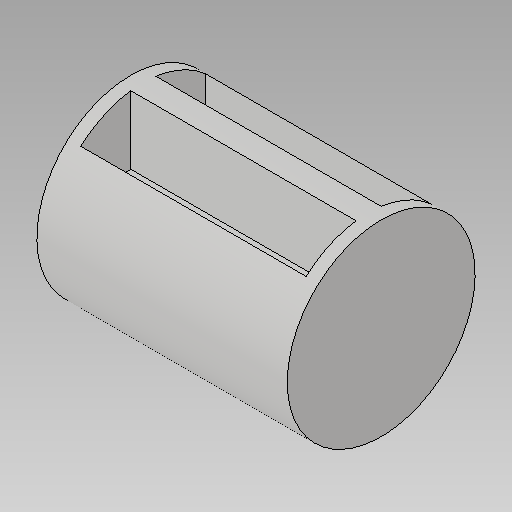
# Autodesk Inventor part: Rounded_beam_body-01
Saved by Autodesk Inventor 2020 (Build 240168000, 168)
## iProperties
Created: 2019-02-05
Part Number: Rounded_beam_body-01
Material: Generic
Document SubType Name: Modeling
Designer: Varga Daniel
Density: 1 g/cm^3
Appearance: Default
Beam_body_length: 10,000 mm
Author: Varga Daniel
Autodesk Inventor part; units mm, degrees
ref_plane "YZ Plane" through (0, 0, 0) normal (1, 0, 0) x (0, 1, 0)
ref_plane "XZ Plane" through (0, 0, 0) normal (0, 1, 0) x (-1, 0, 0)
ref_plane "XY Plane" through (0, 0, 0) normal (0, 0, 1) x (1, 0, 0)
derived "Connector_pin_base.ipt"
sketch "Pin_base_sketch" plane through (0, 0, 0) normal (0, 0, 1) x (1, 0, 0)
  line L0 (0, 0) -> (23.0918, 0) construction
  line L1 (0, 0) -> (0, 6.22) construction
  line L2 (0, 3.75) -> (0.525, 3.75)
  line L3 (0.825, 3.45) -> (0.825, 2.4)
  line L4 (0.825, 2.4) -> (9.225, 2.4)
  line L5 (0, 0) -> (0, 3.75)
  line L6 (0, 0) -> (3.25, 0)
  arc A0 (0.825, 3.45) -> (0.525, 3.75) centre (0.525, 3.45) ccw
  line L7 (0.825, 2.4) -> (0.825, 0.575)
  line L8 (0, 0) -> (-23.0918, 0) construction
  line L9 (9.225, 2.4) -> (9.225, 0.575)
  line L10 (10.025, 2.4) -> (10.025, 2.1865) construction
  line L11 (9.225, 2.4) -> (10.025, 2.4) construction
  line L12 (9.625, 2.4) -> (9.625, 0) construction
  line L13 (10.1291, 2.615) -> (7.4184, 2.615) construction
  line L14 (10.025, 0.575) -> (9.225, 0.575) construction
  line L15 (10.025, 0.575) -> (10.025, 0)
  arc A1 (7.1, 0.575) -> (6.525, 0) centre (7.1, 0) ccw construction
  line L16 (9.225, 0.575) -> (7.1, 0.575) construction
  line L17 (9.225, 0.575) -> (9.225, 0)
  line L18 (0, 0.575) -> (0.825, 0.575) construction
  arc A2 (3.25, 0) -> (2.675, 0.575) centre (2.675, 0) ccw construction
  line L19 (0.825, 0.575) -> (0.825, 0)
  line L20 (0.825, 0.575) -> (2.675, 0.575) construction
  line L21 (0, 0) -> (-3.25, 0)
  line L22 (0, 3.75) -> (-0.525, 3.75)
  line L23 (-0.825, 3.45) -> (-0.825, 2.4)
  arc A3 (-0.525, 3.75) -> (-0.825, 3.45) centre (-0.525, 3.45) ccw
  line L24 (-0.825, 2.4) -> (-0.825, 0.575)
  line L25 (-0.825, 0.575) -> (-0.825, 0)
  line L26 (0, 0.575) -> (-0.825, 0.575) construction
  line L27 (-0.825, 2.4) -> (-9.225, 2.4)
  line L28 (-9.225, 2.4) -> (-9.225, 0)
  line L29 (-10.875, 2.4) -> (-10.875, 0)
  line L30 (-10.5179, 2.55) -> (-9.5821, 2.55)
  line L31 (-10.05, 2.55) -> (-10.05, 0) construction
  line L32 (-9.225, 2.4) -> (-10.875, 2.4) construction
  arc A4 (-10.5179, 2.55) -> (-10.875, 2.4) centre (-10.5179, 2.05) ccw
  arc A5 (-9.225, 2.4) -> (-9.5821, 2.55) centre (-9.5821, 2.05) ccw
  line L33 (-10.875, 2.4) -> (-19.275, 2.4)
  line L34 (-19.275, 2.4) -> (-19.275, 0)
  line L35 (-19.275, 0) -> (-16.575, 0)
  line L36 (-19.275, 2.4) -> (-20.075, 2.4) construction
  line L37 (-20.075, 2.4) -> (-20.075, 2.1865) construction
  line L38 (-20.075, 0) -> (-19.275, 0)
  line L39 (-19.675, 2.4) -> (-19.675, 0) construction
  line L40 (-19.6465, 2.615) -> (-17.4324, 2.615) construction
  line L41 (-0.825, 0.575) -> (-2.675, 0.575) construction
  arc A6 (-2.675, 0.575) -> (-3.25, 0) centre (-2.675, 0) ccw construction
  line L42 (-12.725, 0.575) -> (-7.375, 0.575) construction
  arc A7 (-6.8, 0) -> (-7.375, 0.575) centre (-7.375, 0) ccw construction
  arc A8 (-12.725, 0.575) -> (-13.3, 0) centre (-12.725, 0) ccw construction
  line L43 (-20.075, 0.575) -> (-17.15, 0.575) construction
  arc A9 (-16.575, 0) -> (-17.15, 0.575) centre (-17.15, 0) ccw construction
  line L44 (-16.575, 0) -> (-13.3, 0)
  line L45 (-20.075, 0.575) -> (-20.075, 0)
  line L46 (-13.3, 0) -> (-10.875, 0)
  line L47 (-6.8, 0) -> (-10.875, 0)
  line L48 (-3.25, 0) -> (-6.8, 0)
  line L49 (3.25, 0) -> (6.525, 0)
  line L50 (6.525, 0) -> (10.025, 0)
  arc A10 (-17.15, -0.575) -> (-16.575, 0) centre (-17.15, 0) ccw construction
  line L51 (-20.075, -0.575) -> (-20.075, 0) construction
  line L52 (-20.075, -0.575) -> (-17.15, -0.575) construction
  line L53 (-12.725, -0.575) -> (-7.375, -0.575) construction
  arc A11 (-13.3, 0) -> (-12.725, -0.575) centre (-12.725, 0) ccw construction
  arc A12 (-7.375, -0.575) -> (-6.8, 0) centre (-7.375, 0) ccw construction
  arc A13 (-3.25, 0) -> (-2.675, -0.575) centre (-2.675, 0) ccw construction
  line L54 (-0.825, -0.575) -> (-2.675, -0.575) construction
  line L55 (0, -0.575) -> (-0.825, -0.575) construction
  line L56 (0, -0.575) -> (0.825, -0.575) construction
  line L57 (0.825, -0.575) -> (2.675, -0.575) construction
  arc A14 (2.675, -0.575) -> (3.25, 0) centre (2.675, 0) ccw construction
  arc A15 (6.525, 0) -> (7.1, -0.575) centre (7.1, 0) ccw construction
  line L58 (9.225, -0.575) -> (7.1, -0.575) construction
  line L59 (10.025, -0.575) -> (9.225, -0.575) construction
  line L60 (10.025, -0.575) -> (10.025, 0) construction
  line L61 (-0.025, 0) -> (-0.025, 4.3146) construction
  line L62 (0.025, 0) -> (0.025, 4.3146) construction
  line L63 (-10.075, 0) -> (-10.075, 4.2477) construction
  line L64 (-10.025, 0) -> (-10.025, 4.2339) construction
  arc A16 (-19.275, 2.4) -> (-20.075, 2.1865) centre (-19.6465, 2.1865) ccw
  line L65 (-20.075, 2.1865) -> (-20.075, 0.575)
  arc A17 (10.025, 2.1865) -> (9.225, 2.4) centre (9.5965, 2.1865) ccw
  line L66 (10.025, 2.1865) -> (10.025, 0.575)
derived "Base_part.ipt"
sketch "Sketch3" plane through (0, 0, 0) normal (1, 0, 0) x (0, 1, 0)
  circle A0 centre (0, 0) radius 3.75
  dimension "d1" = 7.5
  constraints: 1 centre point, 1 coincident
  measures "d1" diameter of A0
extrude "Extrusion1" add sketch "Sketch3" along normal blind 10
sketch "Sketch4" plane through (0, 0, 0) normal (0, 1, 0) x (-1, 0, 0)
  line L0 (0, 0) -> (-73.1618, 0) construction
  line L1 (-10, 3.75) -> (-10, -3.75) construction
  line L2 (-0.5, -2.5) -> (-9.5, -2.5)
  line L3 (-9.5, -2.5) -> (-9.5, -0.5)
  line L4 (-9.5, -0.5) -> (-0.5, -0.5)
  line L5 (-0.5, -0.5) -> (-0.5, -2.5)
  line L6 (0, 0) -> (0, -9.7863) construction
  line L7 (-0.5, 2.5) -> (-9.5, 2.5)
  line L8 (-9.5, 2.5) -> (-9.5, 0.5)
  line L9 (-9.5, 0.5) -> (-0.5, 0.5)
  line L10 (-0.5, 0.5) -> (-0.5, 2.5)
  line L11 (-9.6324, -3.6841) -> (-9.6324, 3.75) construction
  line L12 (0, 3.75) -> (-10, 3.75) construction
  dimension "d4" = 0.5
  dimension "d5" = 2
  dimension "d6" = 9
  dimension "d15" = 0.5
  constraints: 22 end point, 4 symmetric about line, 3 perpendicular, 2 parallel, 1 horizontal, 1 point on line
  measures "d4" distance between parallel lines of L0 L4
  measures "d5" distance between parallel lines of L4 L2
  measures "d6" distance between parallel lines of L3 L5
  measures "d15" distance between parallel lines of L6 L5
extrude "Extrusion2" cut sketch "Sketch4" along normal through all both and the other way through all
extrude "Extrusion3" add sketch "Sketch4" along normal mid plane 2
equation "\"d1\" = Base_collar_diameter"
equation "\"d2\" = Beam_body_length"
equation "\"Beam_body_length\" = Body_count"
equation "\"Base_collar_diameter\" = 7.5"
equation "\"Body_count\" = 1"
body "Solid1"
